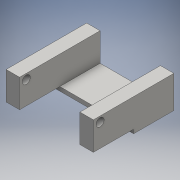
# Autodesk Inventor part: vacuum_cup_base
Saved by Autodesk Inventor 2016 (Build 200138000, 138)
## iProperties
Created: 2016-06-09
Part Number: vacuum_cup_base
Material: 一般
Document SubType Name: Modeling
Designer: Shun Hasegawa
Density: 1 g/cm^3
Appearance: 既定
Author: Shun Hasegawa
Autodesk Inventor part; units mm, degrees
ref_plane "YZ Plane" through (0, 0, 0) normal (1, 0, 0) x (0, 1, 0)
ref_plane "XZ Plane" through (0, 0, 0) normal (0, 1, 0) x (-1, 0, 0)
ref_plane "XY Plane" through (0, 0, 0) normal (0, 0, 1) x (1, 0, 0)
sketch "スケッチ1" plane through (0, 0, 0) normal (0, 0, 1) x (1, 0, 0)
  line L0 (-32.5, 15) -> (32.5, 15)
  line L1 (32.5, 15) -> (32.5, -15)
  line L2 (32.5, -15) -> (-32.5, -15)
  line L3 (-32.5, -15) -> (-32.5, 15)
  line L4 (-45.5, 0) -> (45.5, 0) projected
  line L5 (0, 21) -> (0, -21) projected
  point P0 (0, 0)
  dimension "d0" = 30
  dimension "d1" = 65
  constraints: 8 end point, 2 parallel, 1 horizontal, 1 perpendicular, 2 other
  measures "d0" distance of L0.end L1.end
  measures "d1" distance of L0.start L0.end
extrude "押し出し1" add sketch "スケッチ1" along normal blind 3
sketch "スケッチ2" plane through (0, 0, 3) normal (0, 0, 1) x (1, 0, 0)
  line L0 (32.5, 15) -> (-32.5, 15) projected
  line L1 (-32.5, 15) -> (-22.5, 15)
  line L2 (-22.5, 15) -> (-22.5, -45)
  line L3 (-22.5, -45) -> (-32.5, -45)
  line L4 (-32.5, -45) -> (-32.5, 15)
  line L5 (32.5, -15) -> (32.5, 15) projected
  line L6 (32.5, 15) -> (22.5, 15)
  line L7 (22.5, 15) -> (22.5, -45)
  line L8 (22.5, -45) -> (32.5, -45)
  line L9 (32.5, -45) -> (32.5, 15)
  point P0 (0, 0)
  dimension "d4" = 60
  dimension "d5" = 10
  constraints: 16 end point, 4 parallel, 2 horizontal, 2 perpendicular, 1 collinear, 1 point on line
  measures "d4" distance of L8.end L0.start
  measures "d5" distance of L7.end L8.end
extrude "押し出し2" add sketch "スケッチ2" along normal blind 21
sketch "スケッチ3" plane through (32.5, -15, 0) normal (1, 0, 0) x (0, 0, -1)
  circle A0 centre (-20, -25) radius 3
  line L0 (-24, -30) -> (-24, 30) projected
  line L1 (-3, -30) -> (-24, -30) projected
  point P0 (0, 15)
  dimension "d8" = 4
  dimension "d9" = 5
  dimension "d10" = 6
  constraints: 1 centre point
  measures "d8" distance from line of A0.centre L0
  measures "d9" distance from line of L1 A0.centre
  measures "d10" diameter of A0
extrude "押し出し3" cut sketch "スケッチ3" against normal up to surface (65 mm away)
